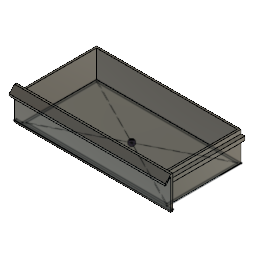
Semana4_Desafio6 (gaveta) v2 (Autodesk Fusion 360 design; units mm, degrees)
Autodesk Fusion 360 part; units mm, degrees
sketch "Sketch1" plane through (0, 0, 0) normal (0, 0, 1) x (1, 0, 0)
  line L0 (185, -95) -> (-185, -95)
  line L1 (-185, -95) -> (-185, 95)
  line L2 (-185, 95) -> (185, 95)
  line L3 (185, 95) -> (185, -95)
  line L4 (185, -95) -> (-185, 95) construction
  line L5 (-185, -95) -> (185, 95) construction
  line L6 (180, -90) -> (-180, -90)
  line L7 (-180, -90) -> (-180, 90)
  line L8 (-180, 90) -> (180, 90)
  line L9 (180, 90) -> (180, -90)
  line L10 (180, -90) -> (-180, 90) construction
  line L11 (-180, -90) -> (180, 90) construction
  line L12 (-185, -95) -> (-200, -95)
  line L13 (-200, -95) -> (-200, -100)
  line L14 (-200, -100) -> (200, -100)
  line L15 (185, -95) -> (200, -95)
  line L16 (200, -95) -> (200, -100)
  dimension "d1" = 370
  dimension "d2" = 190
  dimension "d3" = 360
  dimension "d4" = 180
  dimension "d5" = 400
  dimension "d6" = 15
  dimension "d7" = 5
  constraint horizontal L0
  constraint perpendicular L0 L1
  constraint parallel L0 L2
  constraint parallel L1 L3
  constraint coincident L4 origin
  constraint coincident L5 origin
  constraint horizontal L6
  constraint perpendicular L6 L7
  constraint parallel L6 L8
  constraint parallel L7 L9
  constraint coincident L10 origin
  constraint coincident L11 origin
  constraint perpendicular L1 L12
  constraint perpendicular L12 L13
  constraint perpendicular L13 L14
  constraint perpendicular L3 L15
  constraint perpendicular L14 L16
  measures "d1" distance of L1.end L2.end
  measures "d2" distance of L0.end L1.end
  measures "d3" distance of L7.end L8.end
  measures "d4" distance of L6.end L7.end
  measures "d5" distance of L13.end L14.end
  measures "d6" distance of L0.start L15.end
  measures "d7" distance of L14.end L15.end
extrude "Extrude1" add sketch "Sketch1" along normal blind 75 contours L0 L1 L2 L3
extrude "Extrude2" add sketch "Sketch1" along normal blind 5 contours L6 L7 L8 L9
extrude "Extrude3" add sketch "Sketch1" along normal blind 80 and the other way blind 5 contours L0 L12 L13 L14 L15 L16
sketch "Sketch9" plane through (185, 0, 0) normal (1, 0, 0) x (0, 1, 0)
  line L0 (-95, 0) -> (95, 0)
  line L1 (95, 0) -> (95, 75)
  line L2 (95, 75) -> (-95, 75)
  line L3 (-95, 75) -> (-95, 0)
  line L4 (0, 0) -> (0, 60) construction
  line L5 (0, 60) -> (95, 60) construction
  line L6 (0, 60) -> (-95, 60) construction
  line L7 (-95, 60) -> (95, 60)
  line L8 (95, 60) -> (95, 65)
  line L9 (95, 65) -> (-95, 65)
  line L10 (-95, 65) -> (-95, 60)
  dimension "d48" = 5
  dimension "d49" = 60
  constraint coincident L4.start origin
  constraint perpendicular L0 L4
  constraint coincident L1 L5.end
  constraint perpendicular L1 L5
  constraint coincident L3 L6.end
  constraint perpendicular L3 L6
  constraint horizontal L7
  constraint vertical L8
  constraint horizontal L9
  constraint vertical L10
  measures "d48" distance of L6.end L9.end
  measures "d49" distance of L4.start L4.end
extrude "Extrude10" add sketch "Sketch9" along normal blind 10 contours L1 L3 L7 L8 L9 L10
sketch "Sketch10" plane through (0, 0, 60) normal (0, 0, -1) x (1, 0, 0)
  line L0 (185, 95) -> (185, -95)
  line L1 (185, -95) -> (195, -95)
  line L2 (195, -95) -> (195, 95)
  line L3 (195, 95) -> (185, 95)
  line L4 (195, -95) -> (190, -95)
  line L5 (190, -95) -> (190, 95)
  line L6 (190, 95) -> (195, 95)
  line L7 (195, 95) -> (195, -95)
  constraint horizontal L4
  constraint vertical L5
  constraint horizontal L6
  constraint vertical L7
  constraint midpoint L3 L5.end
  constraint coincident L1.end L2.start
extrude "Extrude11" add sketch "Sketch10" along normal blind 5 contours L1 L2 L3 L4 L5 L6 L7
sketch "Sketch11" plane through (-185, 0, 0) normal (-1, 0, 0) x (0, -1, 0)
  line L0 (-95, 0) -> (95, 0)
  line L1 (95, 0) -> (95, 75)
  line L2 (95, 75) -> (-95, 75)
  line L3 (-95, 75) -> (-95, 0)
  line L4 (0, 0) -> (0, 60) construction
  line L5 (95, 60) -> (-95, 60)
  line L6 (-95, 60) -> (-95, 65)
  line L7 (-95, 65) -> (95, 65)
  line L8 (95, 65) -> (95, 60)
  dimension "d54" = 5
  dimension "d55" = 190
  dimension "d56" = 60
  constraint coincident L4.start origin
  constraint perpendicular L0 L4
  constraint horizontal L5
  constraint vertical L6
  constraint horizontal L7
  constraint vertical L8
  constraint coincident L3 L6.end
  constraint coincident L4.end L5
  measures "d54" distance of L5.start L7.end
  measures "d55" distance of L6.end L7.end
  measures "d56" distance of L4.start L4.end
extrude "Extrude12" add sketch "Sketch11" along normal blind 10 contours L1 L3 L5 L6 L7 L8
sketch "Sketch13" plane through (0, 0, 60) normal (0, 0, -1) x (1, 0, 0)
  line L0 (-185, -95) -> (-185, 95)
  line L1 (-185, 95) -> (-195, 95)
  line L2 (-195, 95) -> (-195, -95)
  line L3 (-195, -95) -> (-185, -95)
  line L4 (-190, -95) -> (-195, -95)
  line L5 (-195, -95) -> (-195, 95)
  line L6 (-195, 95) -> (-190, 95)
  line L7 (-190, 95) -> (-190, -95)
  constraint horizontal L4
  constraint vertical L5
  constraint horizontal L6
  constraint vertical L7
  constraint coincident L1.end L2.start
  constraint midpoint L3 L4.start
extrude "Extrude13" add sketch "Sketch13" along normal blind 5 contours L1 L2 L3 L4 L5 L6 L7
sketch "Sketch14" plane through (0, 0, 0) normal (1, 0, 0) x (0, 1, 0)
  line L0 (-100, 80, -200) -> (-100, 80, 200)
  line L1 (-100, 80) -> (-114.1421, 65.8579)
  line L2 (-100, 80) -> (-120, 80) construction
  line L3 (-114.1421, 65.8579) -> (-114.1421, 60.8579)
  line L4 (-100, 80) -> (-100, 75)
  line L5 (-100, 75) -> (-114.1421, 60.8579)
  dimension "d61" = 45
  dimension "d62" = 20
  dimension "d63" = 5
  constraint horizontal L2
  constraint vertical L3
  constraint perpendicular L2 L4
  constraint parallel L1 L5
  measures "d61" angle of L1 L2
  measures "d62" distance of L1.start L1.end
  measures "d63" distance of L1.end L3.end
extrude "Extrude14" add sketch "Sketch14" along normal mid plane 400
